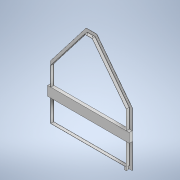
# Autodesk Inventor part: rama podstawa
Saved by Autodesk Inventor 2021 (Build 250183000, 183)
## iProperties
Created: 2022-04-11
Part Number: rama podstawa
Material: Generic
Document SubType Name: Modeling
Designer: Łukasz
Density: 1 g/cm^3
Appearance: Default
Author: Łukasz
Autodesk Inventor part; units mm, degrees
ref_plane "YZ Plane" through (0, 0, 0) normal (1, 0, 0) x (0, 1, 0)
ref_plane "XZ Plane" through (0, 0, 0) normal (0, 1, 0) x (-1, 0, 0)
ref_plane "XY Plane" through (0, 0, 0) normal (0, 0, 1) x (1, 0, 0)
sketch "Sketch1" plane through (0, 0, 0) normal (0, 0, 1) x (1, 0, 0)
  line L0 (0, 0) -> (-1200, 0)
  line L1 (-600, 0) -> (-600, 1500) construction
  line L2 (-600, 0) -> (900, 0) construction
  line L3 (-540, 1500) -> (-660, 1500)
  line L4 (-1200, 0) -> (-1200, 800)
  line L5 (-1200, 0) -> (-400, 0) construction
  line L6 (-1200, 800) -> (-660, 1500)
  line L7 (0, 0) -> (0, 800)
  line L8 (0, 800) -> (-540, 1500)
  dimension "d0" = 1200
  dimension "d1" = 1500
  dimension "d2" = 90
  dimension "d3" = 120
  dimension "d4" = 800
  dimension "d5" = 90
  constraints: 18 end point, 4 horizontal, 3 vertical, 2 perpendicular, 1 midpoint
  measures "d0" distance of L0.start L0.end
  measures "d1" distance of L1.start L1.end
  measures "d2" angle of L2 L1
  measures "d3" distance of L3.start L3.end
  measures "d4" distance of L0.end L4.end
  measures "d5" angle of L5 L4
sketch "Sketch2" plane through (0, 0, 0) normal (0, 1, 0) x (-1, 0, 0)
  line L0 (-3, 0) -> (-50, 0)
  line L1 (0, 3) -> (0, 50) construction
  line L2 (-50, 0) -> (-50, 3)
  line L3 (-50, 3) -> (-6, 3)
  line L4 (-3, 6) -> (-3, 50)
  line L5 (-3, 50) -> (0, 50)
  line L6 (0, 50) -> (0, 0)
  arc A0 (-6, 3) -> (-3, 6) centre (-6, 6) ccw
  arc A1 (-3, 0) -> (0, 3) centre (-3, 3) ccw
  point P0 (-3, 3)
  dimension "d6" = 50
  dimension "d7" = 90
  dimension "d8" = 3
  dimension "d9" = 90
  dimension "d10" = 47
  dimension "d11" = 47
  dimension "d12" = 90
  dimension "d13" = 3
  constraints: 14 end point, 6 perpendicular, 4 point on circle, 4 point on line, 4 tangent, 2 centre point, 1 equal radius
  measures "d6" distance of L6.end L0.end
  measures "d7" angle of L1 L0
  measures "d8" distance of L0.end L2.end
  measures "d9" angle of L0 L2
  measures "d10" distance of L2.end point (-3, 3)
  measures "d11" distance of point (-3, 3) L4.end
  measures "d12" angle of L4 L3
  measures "d13" radius of A0
sweep "Sweep1" add profiles "Sketch2" path "Sketch1" path curves L7 L8 L3 L6 L4 L0
sketch "Sketch3" plane through (-661.4746, 1503, 6) normal (0, 1, 0) x (1, 0, 0)
  circle A0 centre (101.7002, -18.9376) radius 5
  circle A1 centre (21.7002, -18.9376) radius 5
  line L0 (121.7001, -43.9376) -> (121.7001, 3.0624)
  line L1 (121.7001, 3.0624) -> (1.7002, 3.0624)
  line L2 (1.7002, -43.9376) -> (1.7002, 3.0624)
  line L3 (121.7001, -43.9376) -> (1.7002, -43.9376)
  point P0 (661.4746, 6)
  constraints: 8 end point, 2 centre point
extrude "Extrusion1" cut sketch "Sketch3" against normal blind 10 contours A0 | A1
sketch "Sketch4" plane through (-1203, -3, 6) normal (0, -1, 0) x (1, 0, 0)
  line L0 (1206, 0) -> (1206, 44) projected
  line L1 (1206, 44) -> (1176, 44)
  line L2 (1176, 44) -> (1176, 14)
  line L3 (1176, 14) -> (1206, 14)
  line L4 (1206, 14) -> (1206, 44)
  line L5 (1178.5, 41.5) -> (1203.5, 41.5)
  line L6 (1203.5, 41.5) -> (1203.5, 16.5)
  line L7 (1203.5, 16.5) -> (1178.5, 16.5)
  line L8 (1178.5, 16.5) -> (1178.5, 41.5)
  point P0 (1203, -6)
  point P1 (1206, 14)
  dimension "d18" = 30
  dimension "d19" = 30
  dimension "d20" = 25
  dimension "d21" = 25
  dimension "d22" = 2.5
  dimension "d23" = 2.5
  constraints: 16 end point, 4 parallel, 2 horizontal, 2 perpendicular
  measures "d18" distance of L3.end L2.end
  measures "d19" distance of L2.end L1.end
  measures "d20" distance of L6.end L7.end
  measures "d21" distance of L5.end L6.end
  measures "d22" distance between parallel lines of L1 L5
  measures "d23" distance between parallel lines of L2 L8
extrude "Extrusion2" add sketch "Sketch4" along normal blind 50 contours L3 L2 L1 L0 | L5 L6 L7 L8
sketch "Sketch5" plane through (-1203, -53, 6) normal (0, -1, 0) x (1, 0, 0)
  line L0 (1176, 14) -> (1176, 44) construction
  line L1 (1176, 44) -> (1191, 44) construction
  line L2 (1191, 44) -> (1191, 29) construction
  line L3 (1191, 29) -> (1176, 29) construction
  line L4 (1176, 29) -> (1176, 44) construction
  circle A0 centre (1191, 29) radius 4
  point P0 (1203, -6)
  dimension "d26" = 15
  dimension "d27" = 15
  dimension "d28" = 8
  constraints: 8 end point, 2 parallel, 1 centre point, 1 coincident, 1 horizontal, 1 perpendicular
  measures "d26" distance of L2.end L3.end
  measures "d27" distance of L1.end L2.end
  measures "d28" diameter of A0
extrude "Extrusion3" cut sketch "Sketch5" against normal blind 50
sketch "Sketch6" plane through (50, -50, 0) normal (0, 0, -1) x (-1, 0, 0)
  line L0 (1300, 867.0446) -> (1300, 0) projected
  line L1 (0, 0) -> (0, 867.0446) projected
  line L2 (1300, 550) -> (0, 550)
  line L3 (0, 550) -> (0, 400)
  line L4 (0, 400) -> (1300, 400)
  line L5 (1300, 400) -> (1300, 550)
  line L6 (1300, 0) -> (0, 0) projected
  point P0 (50, 50)
  point P1 (0, 550)
  dimension "d31" = 150
  dimension "d32" = 400
  constraints: 8 end point, 2 parallel, 2 point on line, 1 horizontal, 1 perpendicular
  measures "d31" distance of L3.end L2.end
  measures "d32" distance between parallel lines of L6 L4
extrude "Extrusion4" add sketch "Sketch6" against normal blind 50 contours L0 L4 L1 L2
equation "\"d10\" = d6 - d8"
equation "\"d11\" = d6 - d8"
equation "\"d13\" = d8"
equation "\"d23\" = d22"
body "Solid1"
